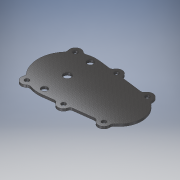
# Autodesk Inventor part: STEEL SIDE REDUCTION COUNTER PLATE
Saved by Autodesk Inventor 2017 (Build 210142000, 142)
## iProperties
Part Number: STEEL SIDE REDUCTION COUNTER PLATE
Material: Genérico
Document SubType Name: Modeling
Designer: Cristian
Density: 1 g/cm^3
Appearance: Valor por defecto
Author: Cristian
Autodesk Inventor part; units mm, degrees
ref_plane "YZ Plane" through (0, 0, 0) normal (1, 0, 0) x (0, 1, 0)
ref_plane "XZ Plane" through (0, 0, 0) normal (0, 1, 0) x (-1, 0, 0)
ref_plane "XY Plane" through (0, 0, 0) normal (0, 0, 1) x (1, 0, 0)
sketch "Boceto1" plane through (0, 0, 0) normal (0, 0, 1) x (1, 0, 0)
  circle A0 centre (0, 0) radius 57.15
  circle A1 centre (101.6, 0) radius 44.45
  circle A2 centre (-31.75, 47.519) radius 11.1125
  circle A3 centre (-31.75, -47.519) radius 11.1125
  circle A4 centre (114.3, 42.5971) radius 11.1125
  circle A5 centre (114.3, -42.5971) radius 11.1125
  line L0 (7.1437, 56.7018) -> (107.1562, 44.1014)
  circle A6 centre (44.45, 52.0016) radius 11.1125
  line L1 (7.1437, -56.7018) -> (107.1562, -44.1014)
  circle A7 centre (44.45, -52.0016) radius 11.1125
  dimension "d0" = 114.3
  dimension "d1" = 88.9
  dimension "d2" = 203.2
  dimension "d3" = 22.225
  dimension "d4" = 22.225
  dimension "d7" = 22.225
  dimension "d8" = 22.225
  dimension "d11" = 22.225
  dimension "d13" = 0
  dimension "d14" = 22.225
  dimension "d27" = 12.7
  dimension "d28" = 12.7
  dimension "d29" = 44.45
  dimension "d30" = 44.45
  dimension "d31" = 31.75
  dimension "d32" = 31.75
  constraints: 8 centre point, 8 point on circle, 4 end point, 4 tangent, 2 point on line, 1 coincident
  measures "d0" diameter of A0
  measures "d1" diameter of A1
  measures "d3" diameter of A2
  measures "d4" diameter of A3
  measures "d7" diameter of A4
  measures "d8" diameter of A5
  measures "d11" diameter of A6
  measures "d13" vertical distance of point (0, 0) A1.centre
  measures "d14" diameter of A7
  measures "d27" horizontal distance of A1.centre A4.centre
  measures "d28" horizontal distance of A1.centre A5.centre
  measures "d29" horizontal distance of point (0, 0) A6.centre
  measures "d30" horizontal distance of A7.centre point (0, 0)
  measures "d31" horizontal distance of point (0, 0) A2.centre
  measures "d32" horizontal distance of point (0, 0) A3.centre
extrude "Extrusión1" add sketch "Boceto1" along normal blind 4.445
sketch "Boceto2" plane through (0, 0, 4.445) normal (0, 0, 1) x (1, 0, 0)
  arc A0 (-21.9537, 52.7651) -> (-40.3458, 40.4764) centre (-31.75, 47.519) ccw projected
  circle A1 centre (-31.75, 47.519) radius 4.2164
  arc A2 (-40.3458, -40.4764) -> (-21.9537, -52.7651) centre (-31.75, -47.519) ccw projected
  circle A3 centre (-31.75, -47.519) radius 4.2164
  arc A4 (33.4247, -53.3907) -> (55.4753, -50.6125) centre (44.45, -52.0016) ccw projected
  circle A5 centre (44.45, -52.0016) radius 4.2164
  arc A6 (55.4753, 50.6125) -> (33.4247, 53.3907) centre (44.45, 52.0016) ccw projected
  circle A7 centre (44.45, 52.0016) radius 4.2164
  arc A8 (124.4689, 38.1158) -> (103.3657, 44.5789) centre (114.3, 42.5971) ccw projected
  circle A9 centre (114.3, 42.5971) radius 4.2164
  arc A10 (103.3657, -44.5789) -> (124.4689, -38.1158) centre (114.3, -42.5971) ccw projected
  circle A11 centre (114.3, -42.5971) radius 4.2164
  point P0 (0, 0)
  dimension "d18" = 8.4328
  dimension "d19" = 8.4328
  dimension "d20" = 8.4328
  dimension "d21" = 8.4328
  dimension "d22" = 8.4328
  dimension "d23" = 8.4328
  constraints: 6 centre point, 6 coincident
  measures "d18" diameter of A1
  measures "d19" diameter of A3
  measures "d20" diameter of A5
  measures "d21" diameter of A7
  measures "d22" diameter of A9
  measures "d23" diameter of A11
extrude "Extrusión2" cut sketch "Boceto2" against normal up to surface (4.445 mm away)
fillet "Empalme1" radius 6.35 12 edges at (-21.9537, -52.7651, 2.2225) (-40.3458, -40.4764, 2.2225) (33.4247, -53.3907, 2.2225) (55.4753, -50.6125, 2.2225) (124.4689, -38.1158, 2.2225) (-40.3458, 40.4764, 2.2225) (-21.9537, 52.7651, 2.2225) (33.4247, 53.3907, 2.2225) (55.4753, 50.6125, 2.2225) (103.3657, 44.5789, 2.2225) (124.4689, 38.1158, 2.2225) (103.3657, -44.5789, 2.2225)
sketch "Boceto3" plane through (0, 0, 0) normal (0, 0, -1) x (-1, 0, 0)
  circle A0 centre (0, 0) radius 7.1437
  circle A1 centre (0, -45) radius 6
  circle A2 centre (0, 45) radius 6
  line L0 (0, -45) -> (0, 0)
  line L1 (0, 0) -> (0, 45)
  dimension "d33" = 14.2875
  dimension "d34" = 12
  dimension "d35" = 12
  dimension "d36" = 45
  dimension "d37" = 45
  constraints: 4 end point, 3 centre point, 1 coincident, 1 collinear, 1 vertical
  measures "d33" diameter of A0
  measures "d34" diameter of A1
  measures "d35" diameter of A2
  measures "d36" distance of point (0, 0) L0.start
  measures "d37" distance of L1.end point (0, 0)
extrude "Extrusión3" cut sketch "Boceto3" against normal up to surface (4.445 mm away)
equation "\"d16\" = t"
equation "\"d18\" = Q"
equation "\"d19\" = Q"
equation "\"d20\" = Q"
equation "\"d21\" = Q"
equation "\"d22\" = Q"
equation "\"d23\" = Q"
equation "\"d33\" = DF"
equation "\"d34\" = NF"
equation "\"d35\" = NF"
equation "\"d36\" = 0.5 * JF"
equation "\"d37\" = 0.5 * JF"
equation "\"t\" = 4.445"
equation "\"Q\" = 8.4328"
equation "\"DF\" = 14.2875"
equation "\"NF\" = 12"
equation "\"JF\" = 90"
